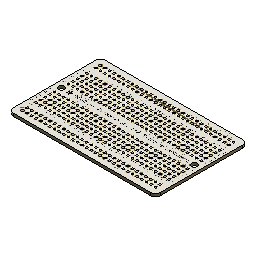
1609 Perma-Proto HalfSize (Autodesk Fusion 360 design; units mm, degrees)
Autodesk Fusion 360 part; units mm, degrees
sketch "sketch 305" plane through (0, 0, 0) normal (0, 0, 1) x (1, 0, 0)
  arc A0 (-38.1, 25.4) -> (-40.64, 22.86) centre (-38.1, 22.86) ccw
  line L0 (-40.64, 22.86) -> (-40.64, -22.86)
  arc A1 (-40.64, -22.86) -> (-38.1, -25.4) centre (-38.1, -22.86) ccw
  line L1 (-38.1, -25.4) -> (38.1, -25.4)
  arc A2 (38.1, -25.4) -> (40.64, -22.86) centre (38.1, -22.86) ccw
  line L2 (40.64, -22.86) -> (40.64, 22.86)
  arc A3 (40.64, 22.86) -> (38.1, 25.4) centre (38.1, 22.86) ccw
  line L3 (38.1, 25.4) -> (-38.1, 25.4)
  circle A4 centre (-36.83, 0) radius 1.6
  circle A5 centre (36.83, 0) radius 1.6
extrude "Board" add sketch "sketch 305" along normal blind 1.57 makes body 1 in component "Board"
sketch "sketch 3085" plane through (0, 0, 0) normal (0, 0, 1) x (1, 0, 0)
  line L0 (-1.342, -1.4015) -> (1.546, -1.4015)
  line L1 (1.546, -1.4015) -> (1.546, 1.4695)
  line L2 (1.546, 1.4695) -> (-1.342, 1.4695)
  line L3 (-1.342, 1.4695) -> (-1.342, -1.4015)
extrude "ADAFRUIT200MIL" add sketch "sketch 3085" along normal blind 0.1 separate body makes body 2 in component "ADAFRUIT200MIL"
sketch "sketch 450" plane through (0, 0, 0) normal (0, 0, 1) x (1, 0, 0)
  circle A0 centre (-36.83, -13.97) radius 0.6
  circle A1 centre (-36.83, -11.43) radius 0.6
  circle A2 centre (-36.83, -8.89) radius 0.6
  circle A3 centre (-36.83, -6.35) radius 0.6
  circle A4 centre (-36.83, -3.81) radius 0.6
  circle A5 centre (-34.29, -13.97) radius 0.6
  circle A6 centre (-34.29, -11.43) radius 0.6
  circle A7 centre (-34.29, -8.89) radius 0.6
  circle A8 centre (-34.29, -6.35) radius 0.6
  circle A9 centre (-34.29, -3.81) radius 0.6
  circle A10 centre (-31.75, -13.97) radius 0.6
  circle A11 centre (-31.75, -11.43) radius 0.6
  circle A12 centre (-31.75, -8.89) radius 0.6
  circle A13 centre (-31.75, -6.35) radius 0.6
  circle A14 centre (-31.75, -3.81) radius 0.6
  circle A15 centre (-29.21, -13.97) radius 0.6
  circle A16 centre (-29.21, -11.43) radius 0.6
  circle A17 centre (-29.21, -8.89) radius 0.6
  circle A18 centre (-29.21, -6.35) radius 0.6
  circle A19 centre (-29.21, -3.81) radius 0.6
  circle A20 centre (-26.67, -13.97) radius 0.6
  circle A21 centre (-26.67, -11.43) radius 0.6
  circle A22 centre (-26.67, -8.89) radius 0.6
  circle A23 centre (-26.67, -6.35) radius 0.6
  circle A24 centre (-26.67, -3.81) radius 0.6
  circle A25 centre (-24.13, -13.97) radius 0.6
  circle A26 centre (-24.13, -11.43) radius 0.6
  circle A27 centre (-24.13, -8.89) radius 0.6
  circle A28 centre (-24.13, -6.35) radius 0.6
  circle A29 centre (-24.13, -3.81) radius 0.6
  circle A30 centre (-19.05, -13.97) radius 0.6
  circle A31 centre (-19.05, -11.43) radius 0.6
  circle A32 centre (-19.05, -8.89) radius 0.6
  circle A33 centre (-19.05, -6.35) radius 0.6
  circle A34 centre (-19.05, -3.81) radius 0.6
  circle A35 centre (-21.59, -13.97) radius 0.6
  circle A36 centre (-21.59, -11.43) radius 0.6
  circle A37 centre (-21.59, -8.89) radius 0.6
  circle A38 centre (-21.59, -6.35) radius 0.6
  circle A39 centre (-21.59, -3.81) radius 0.6
  circle A40 centre (-16.51, -13.97) radius 0.6
  circle A41 centre (-16.51, -11.43) radius 0.6
  circle A42 centre (-16.51, -8.89) radius 0.6
  circle A43 centre (-16.51, -6.35) radius 0.6
  circle A44 centre (-16.51, -3.81) radius 0.6
  circle A45 centre (-13.97, -13.97) radius 0.6
  circle A46 centre (-13.97, -11.43) radius 0.6
  circle A47 centre (-13.97, -8.89) radius 0.6
  circle A48 centre (-13.97, -6.35) radius 0.6
  circle A49 centre (-13.97, -3.81) radius 0.6
  circle A50 centre (-11.43, -13.97) radius 0.6
  circle A51 centre (-11.43, -11.43) radius 0.6
  circle A52 centre (-11.43, -8.89) radius 0.6
  circle A53 centre (-11.43, -6.35) radius 0.6
  circle A54 centre (-11.43, -3.81) radius 0.6
  circle A55 centre (-8.89, -13.97) radius 0.6
  circle A56 centre (-8.89, -11.43) radius 0.6
  circle A57 centre (-8.89, -8.89) radius 0.6
  circle A58 centre (-8.89, -6.35) radius 0.6
  circle A59 centre (-8.89, -3.81) radius 0.6
  circle A60 centre (-6.35, -13.97) radius 0.6
  circle A61 centre (-6.35, -11.43) radius 0.6
  circle A62 centre (-6.35, -8.89) radius 0.6
  circle A63 centre (-6.35, -6.35) radius 0.6
  circle A64 centre (-6.35, -3.81) radius 0.6
  circle A65 centre (-3.81, -13.97) radius 0.6
  circle A66 centre (-3.81, -11.43) radius 0.6
  circle A67 centre (-3.81, -8.89) radius 0.6
  circle A68 centre (-3.81, -6.35) radius 0.6
  circle A69 centre (-3.81, -3.81) radius 0.6
  circle A70 centre (-1.27, -13.97) radius 0.6
  circle A71 centre (-1.27, -11.43) radius 0.6
  circle A72 centre (-1.27, -8.89) radius 0.6
  circle A73 centre (-1.27, -6.35) radius 0.6
  circle A74 centre (-1.27, -3.81) radius 0.6
  circle A75 centre (1.27, -13.97) radius 0.6
  circle A76 centre (1.27, -11.43) radius 0.6
  circle A77 centre (1.27, -8.89) radius 0.6
  circle A78 centre (1.27, -6.35) radius 0.6
  circle A79 centre (1.27, -3.81) radius 0.6
  circle A80 centre (6.35, -13.97) radius 0.6
  circle A81 centre (6.35, -11.43) radius 0.6
  circle A82 centre (6.35, -8.89) radius 0.6
  circle A83 centre (6.35, -6.35) radius 0.6
  circle A84 centre (6.35, -3.81) radius 0.6
  circle A85 centre (3.81, -13.97) radius 0.6
  circle A86 centre (3.81, -11.43) radius 0.6
  circle A87 centre (3.81, -8.89) radius 0.6
  circle A88 centre (3.81, -6.35) radius 0.6
  circle A89 centre (3.81, -3.81) radius 0.6
  circle A90 centre (8.89, -13.97) radius 0.6
  circle A91 centre (8.89, -11.43) radius 0.6
  circle A92 centre (8.89, -8.89) radius 0.6
  circle A93 centre (8.89, -6.35) radius 0.6
  circle A94 centre (8.89, -3.81) radius 0.6
  circle A95 centre (11.43, -13.97) radius 0.6
  circle A96 centre (11.43, -11.43) radius 0.6
  circle A97 centre (11.43, -8.89) radius 0.6
  circle A98 centre (11.43, -6.35) radius 0.6
  circle A99 centre (11.43, -3.81) radius 0.6
  circle A100 centre (16.51, -13.97) radius 0.6
  circle A101 centre (16.51, -11.43) radius 0.6
  circle A102 centre (16.51, -8.89) radius 0.6
  circle A103 centre (16.51, -6.35) radius 0.6
  circle A104 centre (16.51, -3.81) radius 0.6
  circle A105 centre (13.97, -13.97) radius 0.6
  circle A106 centre (13.97, -11.43) radius 0.6
  circle A107 centre (13.97, -8.89) radius 0.6
  circle A108 centre (13.97, -6.35) radius 0.6
  circle A109 centre (13.97, -3.81) radius 0.6
  circle A110 centre (19.05, -13.97) radius 0.6
  circle A111 centre (19.05, -11.43) radius 0.6
  circle A112 centre (19.05, -8.89) radius 0.6
  circle A113 centre (19.05, -3.81) radius 0.6
  circle A114 centre (19.05, -6.35) radius 0.6
  circle A115 centre (21.59, -13.97) radius 0.6
  circle A116 centre (21.59, -11.43) radius 0.6
  circle A117 centre (21.59, -8.89) radius 0.6
  circle A118 centre (21.59, -6.35) radius 0.6
  circle A119 centre (21.59, -3.81) radius 0.6
  circle A120 centre (24.13, -13.97) radius 0.6
  circle A121 centre (24.13, -11.43) radius 0.6
  circle A122 centre (24.13, -8.89) radius 0.6
  circle A123 centre (24.13, -6.35) radius 0.6
  circle A124 centre (24.13, -3.81) radius 0.6
  circle A125 centre (26.67, -13.97) radius 0.6
  circle A126 centre (26.67, -11.43) radius 0.6
  circle A127 centre (26.67, -8.89) radius 0.6
  circle A128 centre (26.67, -6.35) radius 0.6
  circle A129 centre (26.67, -3.81) radius 0.6
  circle A130 centre (31.75, -13.97) radius 0.6
  circle A131 centre (31.75, -11.43) radius 0.6
  circle A132 centre (31.75, -8.89) radius 0.6
  circle A133 centre (31.75, -6.35) radius 0.6
  circle A134 centre (31.75, -3.81) radius 0.6
  circle A135 centre (29.21, -13.97) radius 0.6
  circle A136 centre (29.21, -11.43) radius 0.6
  circle A137 centre (29.21, -8.89) radius 0.6
  circle A138 centre (29.21, -6.35) radius 0.6
  circle A139 centre (29.21, -3.81) radius 0.6
  circle A140 centre (34.29, -13.97) radius 0.6
  circle A141 centre (34.29, -11.43) radius 0.6
  circle A142 centre (34.29, -8.89) radius 0.6
  circle A143 centre (34.29, -6.35) radius 0.6
  circle A144 centre (34.29, -3.81) radius 0.6
  circle A145 centre (36.83, -13.97) radius 0.6
  circle A146 centre (36.83, -11.43) radius 0.6
  circle A147 centre (36.83, -8.89) radius 0.6
  circle A148 centre (36.83, -6.35) radius 0.6
  circle A149 centre (36.83, -3.81) radius 0.6
  circle A150 centre (-36.83, -19.05) radius 0.6
  circle A151 centre (-34.29, -19.05) radius 0.6
  circle A152 centre (-31.75, -19.05) radius 0.6
  circle A153 centre (-29.21, -19.05) radius 0.6
  circle A154 centre (-26.67, -19.05) radius 0.6
  circle A155 centre (-24.13, -19.05) radius 0.6
  circle A156 centre (-21.59, -19.05) radius 0.6
  circle A157 centre (-19.05, -19.05) radius 0.6
  circle A158 centre (-16.51, -19.05) radius 0.6
  circle A159 centre (-13.97, -19.05) radius 0.6
  circle A160 centre (-11.43, -19.05) radius 0.6
  circle A161 centre (-8.89, -19.05) radius 0.6
  circle A162 centre (-6.35, -19.05) radius 0.6
  circle A163 centre (-3.81, -19.05) radius 0.6
  circle A164 centre (-1.27, -19.05) radius 0.6
  circle A165 centre (1.27, -19.05) radius 0.6
  circle A166 centre (3.81, -19.05) radius 0.6
  circle A167 centre (6.35, -19.05) radius 0.6
  circle A168 centre (8.89, -19.05) radius 0.6
  circle A169 centre (11.43, -19.05) radius 0.6
  circle A170 centre (13.97, -19.05) radius 0.6
  circle A171 centre (19.05, -19.05) radius 0.6
  circle A172 centre (16.51, -19.05) radius 0.6
  circle A173 centre (21.59, -19.05) radius 0.6
  circle A174 centre (24.13, -19.05) radius 0.6
  circle A175 centre (26.67, -19.05) radius 0.6
  circle A176 centre (29.21, -19.05) radius 0.6
  circle A177 centre (31.75, -19.05) radius 0.6
  circle A178 centre (34.29, -19.05) radius 0.6
  circle A179 centre (36.83, -19.05) radius 0.6
  circle A180 centre (-36.83, -21.59) radius 0.6
  circle A181 centre (-34.29, -21.59) radius 0.6
  circle A182 centre (-31.75, -21.59) radius 0.6
  circle A183 centre (-29.21, -21.59) radius 0.6
  circle A184 centre (-26.67, -21.59) radius 0.6
  circle A185 centre (-24.13, -21.59) radius 0.6
  circle A186 centre (-21.59, -21.59) radius 0.6
  circle A187 centre (-19.05, -21.59) radius 0.6
  circle A188 centre (-16.51, -21.59) radius 0.6
  circle A189 centre (-13.97, -21.59) radius 0.6
  circle A190 centre (-11.43, -21.59) radius 0.6
  circle A191 centre (-8.89, -21.59) radius 0.6
  circle A192 centre (-6.35, -21.59) radius 0.6
  circle A193 centre (-3.81, -21.59) radius 0.6
  circle A194 centre (-1.27, -21.59) radius 0.6
  circle A195 centre (1.27, -21.59) radius 0.6
  circle A196 centre (3.81, -21.59) radius 0.6
  circle A197 centre (6.35, -21.59) radius 0.6
  circle A198 centre (8.89, -21.59) radius 0.6
  circle A199 centre (11.43, -21.59) radius 0.6
  circle A200 centre (13.97, -21.59) radius 0.6
  circle A201 centre (19.05, -21.59) radius 0.6
  circle A202 centre (16.51, -21.59) radius 0.6
  circle A203 centre (21.59, -21.59) radius 0.6
  circle A204 centre (24.13, -21.59) radius 0.6
  circle A205 centre (26.67, -21.59) radius 0.6
  circle A206 centre (29.21, -21.59) radius 0.6
  circle A207 centre (31.75, -21.59) radius 0.6
  circle A208 centre (34.29, -21.59) radius 0.6
  circle A209 centre (36.83, -21.59) radius 0.6
  circle A210 centre (36.83, 13.97) radius 0.6
  circle A211 centre (36.83, 11.43) radius 0.6
  circle A212 centre (36.83, 8.89) radius 0.6
  circle A213 centre (36.83, 6.35) radius 0.6
  circle A214 centre (36.83, 3.81) radius 0.6
  circle A215 centre (34.29, 13.97) radius 0.6
  circle A216 centre (34.29, 11.43) radius 0.6
  circle A217 centre (34.29, 8.89) radius 0.6
  circle A218 centre (34.29, 6.35) radius 0.6
  circle A219 centre (34.29, 3.81) radius 0.6
  circle A220 centre (31.75, 13.97) radius 0.6
  circle A221 centre (31.75, 11.43) radius 0.6
  circle A222 centre (31.75, 8.89) radius 0.6
  circle A223 centre (31.75, 6.35) radius 0.6
  circle A224 centre (31.75, 3.81) radius 0.6
  circle A225 centre (29.21, 13.97) radius 0.6
  circle A226 centre (29.21, 11.43) radius 0.6
  circle A227 centre (29.21, 8.89) radius 0.6
  circle A228 centre (29.21, 6.35) radius 0.6
  circle A229 centre (29.21, 3.81) radius 0.6
  circle A230 centre (26.67, 13.97) radius 0.6
  circle A231 centre (26.67, 11.43) radius 0.6
  circle A232 centre (26.67, 8.89) radius 0.6
  circle A233 centre (26.67, 6.35) radius 0.6
  circle A234 centre (26.67, 3.81) radius 0.6
  circle A235 centre (24.13, 13.97) radius 0.6
  circle A236 centre (24.13, 11.43) radius 0.6
  circle A237 centre (24.13, 8.89) radius 0.6
  circle A238 centre (24.13, 6.35) radius 0.6
  circle A239 centre (24.13, 3.81) radius 0.6
  circle A240 centre (19.05, 13.97) radius 0.6
  circle A241 centre (19.05, 11.43) radius 0.6
  circle A242 centre (19.05, 8.89) radius 0.6
  circle A243 centre (19.05, 6.35) radius 0.6
  circle A244 centre (19.05, 3.81) radius 0.6
  circle A245 centre (21.59, 13.97) radius 0.6
  circle A246 centre (21.59, 11.43) radius 0.6
  circle A247 centre (21.59, 8.89) radius 0.6
  circle A248 centre (21.59, 6.35) radius 0.6
  circle A249 centre (21.59, 3.81) radius 0.6
  circle A250 centre (16.51, 13.97) radius 0.6
  circle A251 centre (16.51, 11.43) radius 0.6
  circle A252 centre (16.51, 8.89) radius 0.6
  circle A253 centre (16.51, 6.35) radius 0.6
  circle A254 centre (16.51, 3.81) radius 0.6
  circle A255 centre (13.97, 13.97) radius 0.6
  circle A256 centre (13.97, 11.43) radius 0.6
  circle A257 centre (13.97, 8.89) radius 0.6
  circle A258 centre (13.97, 6.35) radius 0.6
  circle A259 centre (13.97, 3.81) radius 0.6
  circle A260 centre (11.43, 13.97) radius 0.6
  circle A261 centre (11.43, 11.43) radius 0.6
  circle A262 centre (11.43, 8.89) radius 0.6
  circle A263 centre (11.43, 6.35) radius 0.6
  circle A264 centre (11.43, 3.81) radius 0.6
  circle A265 centre (8.89, 13.97) radius 0.6
  circle A266 centre (8.89, 11.43) radius 0.6
  circle A267 centre (8.89, 8.89) radius 0.6
  circle A268 centre (8.89, 6.35) radius 0.6
  circle A269 centre (8.89, 3.81) radius 0.6
  circle A270 centre (6.35, 13.97) radius 0.6
  circle A271 centre (6.35, 11.43) radius 0.6
  circle A272 centre (6.35, 8.89) radius 0.6
  circle A273 centre (6.35, 6.35) radius 0.6
  circle A274 centre (6.35, 3.81) radius 0.6
  circle A275 centre (3.81, 13.97) radius 0.6
  circle A276 centre (3.81, 11.43) radius 0.6
  circle A277 centre (3.81, 8.89) radius 0.6
  circle A278 centre (3.81, 6.35) radius 0.6
  circle A279 centre (3.81, 3.81) radius 0.6
  circle A280 centre (1.27, 13.97) radius 0.6
  circle A281 centre (1.27, 11.43) radius 0.6
  circle A282 centre (1.27, 8.89) radius 0.6
  circle A283 centre (1.27, 6.35) radius 0.6
  circle A284 centre (1.27, 3.81) radius 0.6
  circle A285 centre (-1.27, 13.97) radius 0.6
  circle A286 centre (-1.27, 11.43) radius 0.6
  circle A287 centre (-1.27, 8.89) radius 0.6
  circle A288 centre (-1.27, 6.35) radius 0.6
  circle A289 centre (-1.27, 3.81) radius 0.6
  circle A290 centre (-6.35, 13.97) radius 0.6
  circle A291 centre (-6.35, 11.43) radius 0.6
  circle A292 centre (-6.35, 8.89) radius 0.6
  circle A293 centre (-6.35, 6.35) radius 0.6
  circle A294 centre (-6.35, 3.81) radius 0.6
  circle A295 centre (-3.81, 13.97) radius 0.6
  circle A296 centre (-3.81, 11.43) radius 0.6
  circle A297 centre (-3.81, 8.89) radius 0.6
  circle A298 centre (-3.81, 6.35) radius 0.6
  circle A299 centre (-3.81, 3.81) radius 0.6
  circle A300 centre (-8.89, 13.97) radius 0.6
  circle A301 centre (-8.89, 11.43) radius 0.6
  circle A302 centre (-8.89, 8.89) radius 0.6
  circle A303 centre (-8.89, 6.35) radius 0.6
  circle A304 centre (-8.89, 3.81) radius 0.6
  circle A305 centre (-11.43, 13.97) radius 0.6
  circle A306 centre (-11.43, 11.43) radius 0.6
  circle A307 centre (-11.43, 8.89) radius 0.6
  circle A308 centre (-11.43, 6.35) radius 0.6
  circle A309 centre (-11.43, 3.81) radius 0.6
  circle A310 centre (-16.51, 13.97) radius 0.6
  circle A311 centre (-16.51, 11.43) radius 0.6
  circle A312 centre (-16.51, 8.89) radius 0.6
  circle A313 centre (-16.51, 6.35) radius 0.6
  circle A314 centre (-16.51, 3.81) radius 0.6
  circle A315 centre (-13.97, 13.97) radius 0.6
  circle A316 centre (-13.97, 11.43) radius 0.6
  circle A317 centre (-13.97, 8.89) radius 0.6
  circle A318 centre (-13.97, 6.35) radius 0.6
  circle A319 centre (-13.97, 3.81) radius 0.6
  circle A320 centre (-19.05, 13.97) radius 0.6
  circle A321 centre (-19.05, 11.43) radius 0.6
  circle A322 centre (-19.05, 8.89) radius 0.6
  circle A323 centre (-19.05, 3.81) radius 0.6
  circle A324 centre (-19.05, 6.35) radius 0.6
  circle A325 centre (-21.59, 13.97) radius 0.6
  circle A326 centre (-21.59, 11.43) radius 0.6
  circle A327 centre (-21.59, 8.89) radius 0.6
  circle A328 centre (-21.59, 6.35) radius 0.6
  circle A329 centre (-21.59, 3.81) radius 0.6
  circle A330 centre (-24.13, 13.97) radius 0.6
  circle A331 centre (-24.13, 11.43) radius 0.6
  circle A332 centre (-24.13, 8.89) radius 0.6
  circle A333 centre (-24.13, 6.35) radius 0.6
  circle A334 centre (-24.13, 3.81) radius 0.6
  circle A335 centre (-26.67, 13.97) radius 0.6
  circle A336 centre (-26.67, 11.43) radius 0.6
  circle A337 centre (-26.67, 8.89) radius 0.6
  circle A338 centre (-26.67, 6.35) radius 0.6
  circle A339 centre (-26.67, 3.81) radius 0.6
  circle A340 centre (-31.75, 13.97) radius 0.6
  circle A341 centre (-31.75, 11.43) radius 0.6
  circle A342 centre (-31.75, 8.89) radius 0.6
  circle A343 centre (-31.75, 6.35) radius 0.6
  circle A344 centre (-31.75, 3.81) radius 0.6
  circle A345 centre (-29.21, 13.97) radius 0.6
  circle A346 centre (-29.21, 11.43) radius 0.6
  circle A347 centre (-29.21, 8.89) radius 0.6
  circle A348 centre (-29.21, 6.35) radius 0.6
  circle A349 centre (-29.21, 3.81) radius 0.6
  circle A350 centre (-34.29, 13.97) radius 0.6
  circle A351 centre (-34.29, 11.43) radius 0.6
  circle A352 centre (-34.29, 8.89) radius 0.6
  circle A353 centre (-34.29, 6.35) radius 0.6
  circle A354 centre (-34.29, 3.81) radius 0.6
  circle A355 centre (-36.83, 13.97) radius 0.6
  circle A356 centre (-36.83, 11.43) radius 0.6
  circle A357 centre (-36.83, 8.89) radius 0.6
  circle A358 centre (-36.83, 6.35) radius 0.6
  circle A359 centre (-36.83, 3.81) radius 0.6
  circle A360 centre (36.83, 19.05) radius 0.6
  circle A361 centre (34.29, 19.05) radius 0.6
  circle A362 centre (31.75, 19.05) radius 0.6
  circle A363 centre (29.21, 19.05) radius 0.6
  circle A364 centre (26.67, 19.05) radius 0.6
  circle A365 centre (24.13, 19.05) radius 0.6
  circle A366 centre (21.59, 19.05) radius 0.6
  circle A367 centre (19.05, 19.05) radius 0.6
  circle A368 centre (16.51, 19.05) radius 0.6
  circle A369 centre (13.97, 19.05) radius 0.6
  circle A370 centre (11.43, 19.05) radius 0.6
  circle A371 centre (8.89, 19.05) radius 0.6
  circle A372 centre (6.35, 19.05) radius 0.6
  circle A373 centre (3.81, 19.05) radius 0.6
  circle A374 centre (1.27, 19.05) radius 0.6
  circle A375 centre (-1.27, 19.05) radius 0.6
  circle A376 centre (-3.81, 19.05) radius 0.6
  circle A377 centre (-6.35, 19.05) radius 0.6
  circle A378 centre (-8.89, 19.05) radius 0.6
  circle A379 centre (-11.43, 19.05) radius 0.6
  circle A380 centre (-13.97, 19.05) radius 0.6
  circle A381 centre (-19.05, 19.05) radius 0.6
  circle A382 centre (-16.51, 19.05) radius 0.6
  circle A383 centre (-21.59, 19.05) radius 0.6
  circle A384 centre (-24.13, 19.05) radius 0.6
  circle A385 centre (-26.67, 19.05) radius 0.6
  circle A386 centre (-29.21, 19.05) radius 0.6
  circle A387 centre (-31.75, 19.05) radius 0.6
  circle A388 centre (-34.29, 19.05) radius 0.6
  circle A389 centre (-36.83, 19.05) radius 0.6
  circle A390 centre (36.83, 21.59) radius 0.6
  circle A391 centre (34.29, 21.59) radius 0.6
  circle A392 centre (31.75, 21.59) radius 0.6
  circle A393 centre (29.21, 21.59) radius 0.6
  circle A394 centre (26.67, 21.59) radius 0.6
  circle A395 centre (24.13, 21.59) radius 0.6
  circle A396 centre (21.59, 21.59) radius 0.6
  circle A397 centre (19.05, 21.59) radius 0.6
  circle A398 centre (16.51, 21.59) radius 0.6
  circle A399 centre (13.97, 21.59) radius 0.6
  circle A400 centre (11.43, 21.59) radius 0.6
  circle A401 centre (8.89, 21.59) radius 0.6
  circle A402 centre (6.35, 21.59) radius 0.6
  circle A403 centre (3.81, 21.59) radius 0.6
  circle A404 centre (1.27, 21.59) radius 0.6
  circle A405 centre (-1.27, 21.59) radius 0.6
  circle A406 centre (-3.81, 21.59) radius 0.6
  circle A407 centre (-6.35, 21.59) radius 0.6
  circle A408 centre (-8.89, 21.59) radius 0.6
  circle A409 centre (-11.43, 21.59) radius 0.6
  circle A410 centre (-13.97, 21.59) radius 0.6
  circle A411 centre (-19.05, 21.59) radius 0.6
  circle A412 centre (-16.51, 21.59) radius 0.6
  circle A413 centre (-21.59, 21.59) radius 0.6
  circle A414 centre (-24.13, 21.59) radius 0.6
  circle A415 centre (-26.67, 21.59) radius 0.6
  circle A416 centre (-29.21, 21.59) radius 0.6
  circle A417 centre (-31.75, 21.59) radius 0.6
  circle A418 centre (-34.29, 21.59) radius 0.6
  circle A419 centre (-36.83, 21.59) radius 0.6
extrude "Extrude2" cut sketch "sketch 450" along normal blind 1.57 bodies 1 in component "Board"
component "PCB Component" placed x (1, 0, 0) y (0, 1, 0) z (0, 0, 1) at (0, 0, 0)
component "Board" placed x (1, 0, 0) y (0, 1, 0) z (0, 0, 1) at (0, 0, 0) in component "PCB Component"
component "ADAFRUIT200MIL" placed x (0, -1, 0) y (1, 0, 0) z (0, 0, 1) at (-32.258, 0.254, 1.57) in component "PCB Component"
named bodies: "Board", "ADAFRUIT200MIL"
